Autodesk Inventor part; units mm, degrees
(part 2 of 2)
  arc A140 (-25.4446, 74.7133) -> (-26.798, 74.2336) centre (-25.1834, 71.8276) ccw
  arc A141 (-26.798, 74.2336) -> (-27.2062, 73.5932) centre (-26.3001, 73.4659) ccw
  arc A142 (-21.4794, 73.1947) -> (-22.0085, 74.2336) centre (-22.7699, 73.1916) ccw
  circle A143 centre (-25.9605, 73.338) radius 0.5161
  line L110 (-27.2062, 73.5932) -> (-27.2062, 72.1245)
  line L111 (-27.2062, 72.1245) -> (-24.3395, 72.1245)
  line L112 (-24.3395, 71.7056) -> (-28.3839, 71.7056)
  line L113 (-24.3395, 72.1245) -> (-24.3395, 71.7056)
  line L114 (-21.4733, 70.5884) -> (-21.4794, 73.1947)
  arc A144 (-23.3243, 25.8454) -> (-25.4322, 25.8454) centre (-24.3782, 17.6506) ccw
  arc A145 (-25.4322, 25.8454) -> (-26.7856, 25.3656) centre (-25.171, 22.9597) ccw
  arc A146 (-21.9961, 25.3656) -> (-23.3243, 25.8454) centre (-23.7019, 22.7218) ccw
  arc A147 (-21.4671, 24.3267) -> (-21.9961, 25.3656) centre (-22.7575, 24.3237) ccw
  arc A148 (-26.7856, 25.3656) -> (-27.1938, 24.7252) centre (-26.2877, 24.5979) ccw
  circle A149 centre (-25.9607, 24.5305) radius 0.545
  line L115 (-27.1938, 24.7252) -> (-27.1938, 23.2566)
  line L116 (-27.1938, 23.2566) -> (-24.3272, 23.2566)
  line L117 (-24.3272, 23.2566) -> (-24.3272, 22.8376)
  line L118 (-21.461, 21.7204) -> (-21.4671, 24.3267)
  line L119 (-26.0801, 20.1743) -> (-23.0926, 20.1813)
  arc A150 (-22.5618, 19.8544) -> (-21.3196, 20.5365) centre (-22.5875, 21.3734) ccw
  arc A151 (-23.0926, 20.1813) -> (-21.461, 21.7204) centre (-22.9431, 21.6573) ccw
  line L120 (-22.5618, 19.8544) -> (-25.5493, 19.8474)
  line L121 (-21.0597, 22.9429) -> (-21.0597, 21.4689)
  arc A152 (-21.3196, 20.5365) -> (-21.0597, 21.4689) centre (-22.9439, 21.4916) ccw
  line L122 (-19.9288, 22.9429) -> (-21.0597, 22.9429)
  arc A153 (-18.7198, 21.9341) -> (-19.9288, 22.9429) centre (-20.2582, 21.3193) ccw
  arc A154 (-18.5273, 18.7011) -> (-18.7198, 21.9341) centre (-23.4893, 20.0279) ccw
  arc A155 (-20.2704, 17.1911) -> (-18.5273, 18.7011) centre (-20.3549, 19.0497) ccw
  arc A156 (-25.5493, 19.8474) -> (-27.181, 18.3083) centre (-25.6988, 18.3715) ccw
  arc A157 (-26.0801, 20.1743) -> (-27.3224, 19.4922) centre (-26.0545, 18.6554) ccw
  line L123 (-24.3272, 22.8376) -> (-28.3715, 22.8376)
  arc A158 (-27.3224, 19.4922) -> (-27.5822, 18.5598) centre (-25.698, 18.5371) ccw
  line L124 (-27.5822, 17.0858) -> (-27.5822, 18.5598)
  arc A159 (-28.3715, 22.8376) -> (-30.1146, 21.3277) centre (-28.287, 20.979) ccw
  line L125 (-28.7131, 17.0858) -> (-27.5822, 17.0858)
  arc A160 (-30.1146, 21.3277) -> (-29.9221, 18.0946) centre (-25.1526, 20.0009) ccw
  arc A161 (-29.9221, 18.0946) -> (-28.7131, 17.0858) centre (-28.3837, 18.7095) ccw
  arc A162 (-25.3176, 14.1834) -> (-23.2097, 14.1834) centre (-24.2637, 22.3782) ccw
  arc A163 (-26.6458, 14.6631) -> (-25.3176, 14.1834) centre (-24.94, 17.307) ccw
  arc A164 (-23.2097, 14.1834) -> (-21.8563, 14.6631) centre (-23.4709, 17.0691) ccw
  arc A165 (-21.8563, 14.6631) -> (-21.4481, 15.3035) centre (-22.3542, 15.4308) ccw
  arc A166 (-27.1749, 15.702) -> (-26.6458, 14.6631) centre (-25.8844, 15.705) ccw
  circle A167 centre (-22.6938, 15.5587) radius 0.5161
  line L126 (-21.4481, 15.3035) -> (-21.4481, 16.7721)
  line L127 (-21.4481, 16.7721) -> (-24.3148, 16.7721)
  line L128 (-24.3148, 17.1911) -> (-20.2704, 17.1911)
  line L129 (-24.3148, 16.7721) -> (-24.3148, 17.1911)
  line L130 (-27.181, 18.3083) -> (-27.1749, 15.702)
  line L131 (-50.2817, 78.9621) -> (-51.492, 78.9621)
  line L132 (-51.492, 78.9621) -> (-51.492, 75.4711)
  line L133 (-51.492, 75.4711) -> (-52.8011, 75.4711)
  line L134 (-52.8011, 75.4711) -> (-52.8011, 78.9621)
  line L135 (-52.8011, 78.9621) -> (-57.2883, 78.9621)
  line L136 (-57.2883, 78.9621) -> (-57.2883, 80.3947)
  line L137 (-57.2883, 80.3947) -> (-52.7435, 85.6311)
  line L138 (-52.7435, 85.6311) -> (-51.492, 85.6311)
  line L139 (-51.492, 85.6311) -> (-51.492, 80.0571)
  line L140 (-51.492, 80.0571) -> (-50.2817, 80.0571)
  line L141 (-50.2817, 80.0571) -> (-50.2817, 78.9621)
  line L142 (-52.8011, 80.0571) -> (-52.8011, 84.0256)
  line L143 (-52.8011, 84.0256) -> (-56.218, 80.0571)
  line L144 (-56.218, 80.0571) -> (-52.8011, 80.0571)
  line L145 (-13.2183, 10.2825) -> (-12.008, 10.2825)
  line L146 (-12.008, 10.2825) -> (-12.008, 13.7735)
  line L147 (-12.008, 13.7735) -> (-10.6989, 13.7735)
  line L148 (-10.6989, 13.7735) -> (-10.6989, 10.2825)
  line L149 (-10.6989, 10.2825) -> (-6.2117, 10.2825)
  line L150 (-6.2117, 10.2825) -> (-6.2117, 8.8499)
  line L151 (-6.2117, 8.8499) -> (-10.7565, 3.6135)
  line L152 (-10.7565, 3.6135) -> (-12.008, 3.6135)
  line L153 (-12.008, 3.6135) -> (-12.008, 9.1875)
  line L154 (-12.008, 9.1875) -> (-13.2183, 9.1875)
  line L155 (-13.2183, 9.1875) -> (-13.2183, 10.2825)
  line L156 (-10.6989, 9.1875) -> (-10.6989, 5.219)
  line L157 (-10.6989, 5.219) -> (-7.282, 9.1875)
  line L158 (-7.282, 9.1875) -> (-10.6989, 9.1875)
  line L159 (-50.2817, 78.9621) -> (-51.492, 78.9621)
  line L160 (-51.492, 78.9621) -> (-51.492, 75.4711)
  line L161 (-51.492, 75.4711) -> (-52.8011, 75.4711)
  line L162 (-52.8011, 75.4711) -> (-52.8011, 78.9621)
  line L163 (-52.8011, 78.9621) -> (-57.2883, 78.9621)
  line L164 (-57.2883, 78.9621) -> (-57.2883, 80.3947)
  line L165 (-57.2883, 80.3947) -> (-52.7435, 85.6311)
  line L166 (-52.7435, 85.6311) -> (-51.492, 85.6311)
  line L167 (-51.492, 85.6311) -> (-51.492, 80.0571)
  line L168 (-51.492, 80.0571) -> (-50.2817, 80.0571)
  line L169 (-50.2817, 80.0571) -> (-50.2817, 78.9621)
  line L170 (-52.8011, 80.0571) -> (-52.8011, 84.0256)
  line L171 (-52.8011, 84.0256) -> (-56.218, 80.0571)
  line L172 (-56.218, 80.0571) -> (-52.8011, 80.0571)
  line L173 (-13.2183, 10.2825) -> (-12.008, 10.2825)
  line L174 (-12.008, 10.2825) -> (-12.008, 13.7735)
  line L175 (-12.008, 13.7735) -> (-10.6989, 13.7735)
  line L176 (-10.6989, 13.7735) -> (-10.6989, 10.2825)
  line L177 (-10.6989, 10.2825) -> (-6.2117, 10.2825)
  line L178 (-6.2117, 10.2825) -> (-6.2117, 8.8499)
  line L179 (-6.2117, 8.8499) -> (-10.7565, 3.6135)
  line L180 (-10.7565, 3.6135) -> (-12.008, 3.6135)
  line L181 (-12.008, 3.6135) -> (-12.008, 9.1875)
  line L182 (-12.008, 9.1875) -> (-13.2183, 9.1875)
  line L183 (-13.2183, 9.1875) -> (-13.2183, 10.2825)
  line L184 (-10.6989, 9.1875) -> (-10.6989, 5.219)
  line L185 (-10.6989, 5.219) -> (-7.282, 9.1875)
  line L186 (-7.282, 9.1875) -> (-10.6989, 9.1875)
  point P0 (-39.1737, 68.8958)
  point P1 (-39.1737, 20.0009)
  point P2 (-53.7479, 68.8958)
  point P3 (-9.7521, 20.0042)
  point P4 (-13.4723, 102.9238)
  point P5 (-39.1737, 68.8958)
  point P6 (-39.1737, 20.0009)
  point P7 (-53.7479, 68.8958)
  point P8 (-9.7521, 20.0042)
  point P9 (-24.3263, 68.8958)
  point P10 (-24.3272, 68.8958)
  point P11 (-24.3272, 20.0009)
  point P12 (-24.3272, 68.8958)
  point P13 (-24.3272, 20.0009)
  dimension "d103" = 8.4153
  dimension "d105" = 0.508
  dimension "d106" = 0.508
  constraints: 308 point on circle, 236 end point, 168 centre point, 28 perpendicular, 28 tangent, 10 vertical, 5 horizontal, 3 midpoint, 1 parallel, 1 symmetric about line, 4 other
  measures "d103" distance of L12.end L14.start
  measures "d105" distance between parallel lines of L15 L7
  measures "d106" distance between parallel lines of L16 L11
extrude "Extrusion20" add sketch "Sketch17" along normal blind 0.4 contours L40 A34 A33 A32 L39 L38 L37 L36 A31 A30 A29 A28 A27 L35 A26 L34 A25 A24 L33 | L56 A58 A57 A56 L55 L54 L53 L52 A55 A54 A53 A52 A51 L51 A50 L50 A49 A48 L49 | L72 A82 A81 A80 L71 L70 L69 L68 A79 A78 A77 A76 A75 L67 A74 L66 A73 A72 L65 | L92 A113 A112 L95 L96 A116 A117 A115 L93 L89 L91 L94 A111 A110 A108 A114 A109 L90 A107 | A122 A123 L102 A127 L103 A133 A134 L108 L109 A137 A136 A135 L107 L101 L100 L99 A124 A121 A120 | A150 A152 L121 L122 A153 A154 A155 L128 L129 L127 L126 A165 A164 A162 A163 A166 L130 A156 L120 | L131 L132 L133 L134 L135 L136 L137 L138 L139 L140 L141 | L145 L146 L147 L148 L149 L150 L151 L152 L153 L154 L155 bodies 1
sketch "Sketch18" plane through (0, 0, -0.2) normal (0, 0, -1) x (-1, 0, 0)
  line L0 (0, 0) -> (-63.5, 0)
  line L1 (-63.5, 0) -> (-63.5, 88.9)
  line L2 (-63.5, 88.9) -> (0, 88.9)
  line L3 (0, 88.9) -> (0, 0)
  constraints: 8 end point, 2 parallel, 1 horizontal, 1 perpendicular
extrude "Extrusion21" add sketch "Sketch18" along normal blind 0.4 bodies 3
fillet "Fillet2" radius 3.175 8 edges at (63.5, 0, 0.2) (63.5, 88.9, 0.2) (0, 0, 0.2) (0, 88.9, 0.2) (63.5, 0, -0.3) (63.5, 88.9, -0.3) (0, 0, -0.3) (0, 88.9, -0.3)
extrude "Extrusion22" cut sketch "Sketch17" along normal blind 0.4 contours L40 A34 A33 A32 L39 L38 L37 L36 A31 A30 A29 A28 A27 L35 A26 L34 A25 A24 L33 | L44 A41 A40 L47 L48 A44 A45 A43 L45 L41 L43 L46 A39 A38 A36 A42 A37 L42 A35 | L56 A58 A57 A56 L55 L54 L53 L52 A55 A54 A53 A52 A51 L51 A50 L50 A49 A48 L49 | L60 A65 A64 L63 L64 A68 A69 A67 L61 L57 L59 L62 A63 A62 A60 A66 A61 L58 A59 | L72 A82 A81 A80 L71 L70 L69 L68 A79 A78 A77 A76 A75 L67 A74 L66 A73 A72 L65 | L76 A89 A88 L79 L80 A92 A93 A91 L77 L73 L75 L78 A87 A86 A84 A90 A85 L74 A83 | L88 A106 A105 A104 L87 L86 L85 L84 A103 A102 A101 A100 A99 L83 A98 L82 A97 A96 L81 | L92 A113 A112 L95 L96 A116 A117 A115 L93 L89 L91 L94 A111 A110 A108 A114 A109 L90 A107 | A122 A123 L102 A127 L103 A133 A134 L108 L109 A137 A136 A135 L107 L101 L100 L99 A124 A121 A120 | A126 A128 L105 L106 A129 A130 A131 L112 L113 L111 L110 A141 A140 A138 A139 A142 L114 A132 L104 | A146 A147 L118 A151 L119 A157 A158 L124 L125 A161 A160 A159 L123 L117 L116 L115 A148 A145 A144 | A150 A152 L121 L122 A153 A154 A155 L128 L129 L127 L126 A165 A164 A162 A163 A166 L130 A156 L120 | L131 L132 L133 L134 L135 L136 L137 L138 L139 L140 L141 | L145 L146 L147 L148 L149 L150 L151 L152 L153 L154 L155 bodies 3
extrude "Extrusion23" add sketch "Sketch17" along normal blind 0.4 contours L44 A41 A40 L47 L48 A44 A45 A43 L45 L41 L43 L46 A39 A38 A36 A42 A37 L42 A35 | L60 A65 A64 L63 L64 A68 A69 A67 L61 L57 L59 L62 A63 A62 A60 A66 A61 L58 A59 | L76 A89 A88 L79 L80 A92 A93 A91 L77 L73 L75 L78 A87 A86 A84 A90 A85 L74 A83 | L88 A106 A105 A104 L87 L86 L85 L84 A103 A102 A101 A100 A99 L83 A98 L82 A97 A96 L81 | A126 A128 L105 L106 A129 A130 A131 L112 L113 L111 L110 A141 A140 A138 A139 A142 L114 A132 L104 | A146 A147 L118 A151 L119 A157 A158 L124 L125 A161 A160 A159 L123 L117 L116 L115 A148 A145 A144 bodies 4
